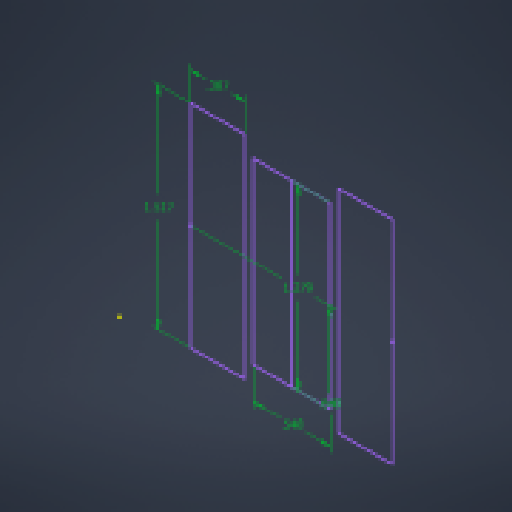
# Autodesk Inventor part: Wheel Bracket
Saved by Autodesk Inventor 2027 (Build 310192000, 192)
## iProperties
Created: 2026-07-06
Part Number: Wheel Bracket
Material: Generic
Document SubType Name: Modeling
Designer: belcz
Density: 1 g/cm^3
Appearance: Default
Author: belcz
Autodesk Inventor part; units mm, degrees
ref_plane "YZ Plane" through (0, 0, 0) normal (1, 0, 0) x (0, 1, 0)
ref_plane "XZ Plane" through (0, 0, 0) normal (0, 1, 0) x (-1, 0, 0)
ref_plane "XY Plane" through (0, 0, 0) normal (0, 0, 1) x (1, 0, 0)
sketch "Sketch1" plane through (0, 0, 0) normal (0, 0, 1) x (1, 0, 0)
  line L0 (38.3225, 4.6263) -> (24.416, 4.6263)
  line L1 (38.3225, 4.6263) -> (38.3225, 37.1129)
  line L2 (38.3225, 37.1129) -> (24.416, 37.1129)
  line L3 (24.416, 37.1129) -> (24.416, 4.6263)
  line L4 (9.8554, 1.6101) -> (9.8554, 40.1292)
  line L5 (9.8554, 40.1292) -> (19.6852, 40.1292)
  line L6 (19.6852, 40.1292) -> (19.6852, 1.6101)
  line L7 (19.6852, 1.6101) -> (9.8554, 1.6101)
  line L8 (31.3692, 4.6263) -> (31.3692, 37.1129)
  line L9 (52.883, 1.6101) -> (52.883, 40.1292)
  line L10 (52.883, 40.1292) -> (43.0532, 40.1292)
  line L11 (43.0532, 40.1292) -> (43.0532, 1.6101)
  line L12 (43.0532, 1.6101) -> (52.883, 1.6101)
  point P0 (0, 0)
  point P1 (9.8554, 20.8696)
  point P2 (52.883, 20.8696)
  dimension "d0" = 13.9065
  dimension "d1" = 32.4866
  dimension "d2" = 38.5191
  dimension "d3" = 16.2433
  dimension "d5" = 9.8298
  dimension "d31" = 43.0276
  dimension "d59" = 38.5191
  constraints: 26 end point, 5 symmetric about line, 4 perpendicular, 3 midpoint, 2 horizontal, 2 vertical
  measures "d0" distance of L0.start L0.end
  measures "d1" distance of L0.start L1.end
  measures "d2" distance of L4.start L4.end
  measures "d3" vertical distance of L8.start point (9.855, 20.87)
  measures "d5" distance of L4.end L5.end
  measures "d31" distance between parallel lines of L4 L9
  measures "d59" distance between parallel lines of L12 L5
extrude "Extrusion6" add sketch "Sketch1" along normal blind 3.048 contours L4 L5 L6 L7 | L12 L11 L10 L9
extrude "Extrusion7" add sketch "Sketch1" along normal blind 10.287 contours L0 L8 L2 L1 | L0 L3 L2 L8
sketch "Sketch6" plane through (24.416, 37.1129, 0) normal (0, 1, 0) x (1, 0, 0)
  line L0 (13.9065, 0) -> (0, 0) projected
  line L1 (0, 0) -> (0, -10.287) projected
  line L2 (13.9065, -10.287) -> (0, -10.287) projected
  line L3 (13.9065, 0) -> (13.9065, -10.287) projected
  line L4 (13.9065, -7.239) -> (0, -7.239)
  point P0 (-24.416, 0)
  dimension "d36" = 3.048
  constraints: 2 end point, 2 point on line, 1 perpendicular
  measures "d36" distance between parallel lines of L2 L4
extrude "Extrusion8" cut sketch "Sketch6" against normal blind 50.8 contours L3 L4 L1 L0
sketch "Sketch7" plane through (24.416, 37.1129, 10.287) normal (0, 1, 0) x (1, 0, 0)
  line L0 (28.4671, 7.239) -> (18.6373, 7.239) projected
  line L1 (0, 0) -> (13.9065, 0) projected
  line L2 (20.4193, 12.3132) -> (10.4121, 0.6025)
  line L3 (23.3323, 11.0303) -> (13.9065, 0)
  line L4 (13.9065, 3.048) -> (13.9065, 0) projected
  line L5 (13.9065, 0) -> (10.4121, 0)
  line L6 (10.4121, 0.6025) -> (10.4121, 0)
  line L7 (28.4671, 10.287) -> (18.6373, 10.287) projected
  line L8 (18.6373, 10.287) -> (18.6373, 7.239) projected
  line L9 (28.4671, 7.239) -> (18.6373, 7.239) projected
  line L10 (28.4671, 10.287) -> (28.4671, 7.239) projected
  line L11 (13.9065, 3.048) -> (0, 3.048) projected
  line L12 (0, 3.048) -> (0, 0) projected
  line L13 (13.9065, 0) -> (0, 0) projected
  line L14 (13.9065, 3.048) -> (13.9065, 0) projected
  line L15 (6.9533, 0) -> (6.9533, 10.1633)
  line L16 (-14.5606, 7.239) -> (-4.7307, 7.239)
  line L17 (-6.5128, 12.3132) -> (3.4944, 0.6025)
  line L18 (-9.4258, 11.0303) -> (0, 0)
  line L19 (0, 0) -> (3.4944, 0)
  line L20 (3.4944, 0.6025) -> (3.4944, 0)
  line L21 (-14.5606, 10.287) -> (-4.7307, 10.287)
  point P0 (-24.416, 10.287)
  point P1 (1.4047, 3.048)
  point P2 (-4.7813, 10.287)
  point P3 (-8.7906, 10.287)
  point P4 (12.5018, 3.048)
  point P5 (20.0925, 7.239)
  point P6 (18.6373, 10.2278)
  dimension "d39" = 3.048
  dimension "d40" = 0
  dimension "d41" = 0
  constraints: 22 end point, 10 symmetric about line, 1 midpoint, 1 parallel, 1 perpendicular, 1 point on line, 1 vertical
  measures "d39" distance between parallel lines of L2 L3
  measures "d40" distance of L1.end L3.end
  measures "d41" distance of L1.end L3.end
extrude "Extrusion9" add sketch "Sketch7" against normal blind 32.4866 contours L3 L4 L11 L2 L8 L0 | L11 L12 L18 L21 L17
sketch "Sketch8" plane through (0, 0, 3.048) normal (0, 0, 1) x (1, 0, 0)
  circle A0 centre (14.6052, 7.9601) radius 3.175
  line L0 (9.8554, 1.6101) -> (19.6852, 1.6101) projected
  circle A1 centre (14.6052, 33.7792) radius 3.175
  line L1 (19.6852, 40.1292) -> (9.8554, 40.1292) projected
  line L2 (38.3225, 37.1129) -> (24.416, 37.1129) projected
  line L3 (24.416, 37.1129) -> (24.416, 4.6263) projected
  line L4 (24.416, 4.6263) -> (38.3225, 4.6263) projected
  line L5 (38.3225, 4.6263) -> (38.3225, 37.1129) projected
  line L6 (38.3225, 37.1129) -> (24.416, 37.1129) projected
  line L7 (31.3692, 37.1129) -> (31.3692, 17.7925)
  line L8 (19.6852, 1.6101) -> (19.6852, 40.1292) projected
  line L9 (19.6852, 1.6101) -> (19.6852, 4.6263) projected
  circle A2 centre (48.1332, 7.9601) radius 3.175
  circle A3 centre (48.1332, 33.7792) radius 3.175
  point P0 (0, 0)
  point P1 (19.6852, 37.1129)
  point P2 (19.6852, 38.6211)
  dimension "d44" = 6.35
  dimension "d45" = 6.35
  dimension "d46" = 6.35
  dimension "d47" = 6.35
  dimension "d55" = 5.08
  dimension "d56" = 5.08
  constraints: 4 centre point, 2 end point, 2 symmetric about line, 1 midpoint, 1 point on line, 1 vertical, 2 other
  measures "d44" diameter of A0
  measures "d45" distance from line of L0 A0.centre
  measures "d46" diameter of A1
  measures "d47" distance from line of L1 A1.centre
  measures "d55" horizontal distance of point (19.685, 38.621) A1.centre
  measures "d56" distance from line of L9 A0.centre
fillet "Fillet4" radius 1.27 12 edges at (9.8554, 40.1292, 1.524) (19.6852, 40.1292, 1.524) (19.6852, 37.1129, 1.5536) (43.0532, 37.1129, 1.5536) (43.0532, 40.1292, 1.524) (52.883, 40.1292, 1.524) (52.883, 1.6101, 1.524) (43.0532, 1.6101, 1.524) (9.8554, 1.6101, 1.524) (19.6852, 1.6101, 1.524) (19.6852, 4.6263, 1.5536) (43.0532, 4.6263, 1.5536)
fillet "Fillet5" radius 6.35 2 edges at (24.416, 20.8696, 10.287) (38.3225, 20.8696, 10.287)
fillet "Fillet6" radius 1.27 1 edges at (18.23, 20.8696, 3.048)
fillet "Fillet7" radius 1.27 1 edges at (44.5085, 20.8696, 3.048)
fillet "Fillet8" radius 1.27 2 edges at (25.8207, 20.8696, 7.239) (36.9178, 20.8696, 7.239)
extrude "Extrusion11" cut sketch "Sketch8" against normal blind 50.8 contours A0 | A1 | A2 | A3
body "Solid2"
